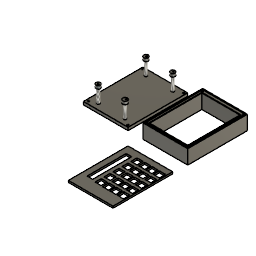
macropad-test-design (Autodesk Fusion 360 archive; units mm, degrees)
design "macropad-test-design"
part number: 2026-08-19-18-04-08-629
Autodesk Fusion 360 part; units mm, degrees
sketch "Sketch1" plane through (0, 0, 0) normal (0, 0, 1) x (1, 0, 0)
  line L0 (0, 100) -> (75, 100)
  line L1 (75, 100) -> (75, 0)
  line L2 (75, 0) -> (0, 0)
  line L3 (0, 0) -> (0, 100)
  line L4 (6.0568, 92.5343) -> (70, 92.5343)
  line L5 (70, 92.5343) -> (70, 5)
  line L6 (70, 5) -> (6.0568, 5)
  line L7 (6.0568, 5) -> (6.0568, 92.5343)
  constraint horizontal L0
  constraint vertical L1
  constraint horizontal L2
  constraint vertical L3
  constraint horizontal L4
  constraint vertical L5
  constraint horizontal L6
  constraint vertical L7
extrude "Extrude1" add sketch "Sketch1" along normal blind 20 makes body 1
sketch "Sketch2" plane through (0, 0, 0) normal (0, 0, 1) x (1, 0, 0)
  line L0 (-100, 100) -> (-25, 100)
  line L1 (-25, 100) -> (-25, 0)
  line L2 (-25, 0) -> (-100, 0)
  line L3 (-100, 0) -> (-100, 100)
  constraint horizontal L0
  constraint vertical L1
  constraint horizontal L2
  constraint vertical L3
extrude "Extrude2" add sketch "Sketch2" along normal blind 5 separate body makes body 2
cylinder "CylinderPrimitive1" add diameter 5 height 23 placed x (1, 0, 0) y (0, 1, 0) z (0, 0, 1) at (-40, 90, 5) bodies 2
cylinder "CylinderPrimitive2" add diameter 5 height 23 placed x (1, 0, 0) y (0, 1, 0) z (0, 0, 1) at (-85, 90, 5) bodies 2
cylinder "CylinderPrimitive3" add diameter 5 height 23 placed x (1, 0, 0) y (0, 1, 0) z (0, 0, 1) at (-85, 10, 5) bodies 2
cylinder "CylinderPrimitive4" add diameter 5 height 23 placed x (1, 0, 0) y (0, 1, 0) z (0, 0, 1) at (-40, 10, 5) bodies 2
extrude "Extrude3" add 1 faces at (27.0189, 97.5114, 20) along direction (0, 0, 1) blind 4 thin wall 1 inside on bodies 1 bodies 1
sketch "Sketch7" plane through (0, 0, 0) normal (0, 0, 1) x (1, 0, 0)
  line L0 (0, -25) -> (75, -25)
  line L1 (75, -25) -> (75, -125.149)
  line L2 (75, -125.149) -> (0, -125.149)
  line L3 (0, -125.149) -> (0, -25)
  constraint horizontal L0
  constraint vertical L1
  constraint horizontal L2
  constraint vertical L3
extrude "Extrude4" add sketch "Sketch7" along normal blind 3 separate body makes body 3
sketch "Sketch8" plane through (0, 0, 3) normal (0, 0, 1) x (-1, 0, 0)
  line L0 (0, 125.149) -> (-75, 125.149)
  line L1 (-75, 125.149) -> (-75, 25)
  line L2 (-75, 25) -> (0, 25)
  line L3 (0, 25) -> (0, 125.149)
  line L4 (-25, 35) -> (-35, 35)
  line L5 (-35, 35) -> (-35, 45)
  line L6 (-35, 45) -> (-25, 45)
  line L7 (-25, 45) -> (-25, 35)
  line L8 (-37.6867, 35) -> (-48.0057, 35)
  line L9 (-48.0057, 35) -> (-48.0057, 45)
  line L10 (-48.0057, 45) -> (-37.6867, 45)
  line L11 (-37.6867, 45) -> (-37.6867, 35)
  line L12 (-50, 35) -> (-60, 35)
  line L13 (-60, 35) -> (-60, 45)
  line L14 (-60, 45) -> (-50, 45)
  line L15 (-50, 45) -> (-50, 35)
  line L16 (-62.3625, 35) -> (-72.6815, 35)
  line L17 (-72.6815, 35) -> (-72.6815, 45)
  line L18 (-72.6815, 45) -> (-62.3625, 45)
  line L19 (-62.3625, 45) -> (-62.3625, 35)
  line L20 (-25, 50) -> (-35, 50)
  line L21 (-35, 50) -> (-35, 60)
  line L22 (-35, 60) -> (-25, 60)
  line L23 (-25, 60) -> (-25, 50)
  line L24 (-37.6867, 50) -> (-48.23, 50)
  line L25 (-48.23, 50) -> (-48.23, 60)
  line L26 (-48.23, 60) -> (-37.6867, 60)
  line L27 (-37.6867, 60) -> (-37.6867, 50)
  line L28 (-50, 50) -> (-60, 50)
  line L29 (-60, 50) -> (-60, 60)
  line L30 (-60, 60) -> (-50, 60)
  line L31 (-50, 60) -> (-50, 50)
  line L32 (-62.8111, 50) -> (-72.6815, 50)
  line L33 (-72.6815, 50) -> (-72.6815, 59.3341)
  line L34 (-72.6815, 59.3341) -> (-62.8111, 59.3341)
  line L35 (-62.8111, 59.3341) -> (-62.8111, 50)
  line L36 (-25, 65) -> (-35, 65)
  line L37 (-35, 65) -> (-35, 75)
  line L38 (-35, 75) -> (-25, 75)
  line L39 (-25, 75) -> (-25, 65)
  line L40 (-38.1353, 65) -> (-48.23, 65)
  line L41 (-48.23, 65) -> (-48.23, 75)
  line L42 (-48.23, 75) -> (-38.1353, 75)
  line L43 (-38.1353, 75) -> (-38.1353, 65)
  line L44 (-50, 65) -> (-60, 65)
  line L45 (-60, 65) -> (-60, 75)
  line L46 (-60, 75) -> (-50, 75)
  line L47 (-50, 75) -> (-50, 65)
  line L48 (-62.5868, 65) -> (-72.9058, 65)
  line L49 (-72.9058, 65) -> (-72.9058, 75)
  line L50 (-72.9058, 75) -> (-62.5868, 75)
  line L51 (-62.5868, 75) -> (-62.5868, 65)
  line L52 (-25, 80) -> (-35, 80)
  line L53 (-35, 80) -> (-35, 90)
  line L54 (-35, 90) -> (-25, 90)
  line L55 (-25, 90) -> (-25, 80)
  line L56 (-38.1353, 80) -> (-48.23, 80)
  line L57 (-48.23, 80) -> (-48.23, 90)
  line L58 (-48.23, 90) -> (-38.1353, 90)
  line L59 (-38.1353, 90) -> (-38.1353, 80)
  line L60 (-50, 80) -> (-60, 80)
  line L61 (-60, 80) -> (-60, 90)
  line L62 (-60, 90) -> (-50, 90)
  line L63 (-50, 90) -> (-50, 80)
  line L64 (-62.3625, 80) -> (-72.9058, 80)
  line L65 (-72.9058, 80) -> (-72.9058, 90)
  line L66 (-72.9058, 90) -> (-62.3625, 90)
  line L67 (-62.3625, 90) -> (-62.3625, 80)
  line L68 (-25, 95) -> (-35, 95)
  line L69 (-35, 95) -> (-35, 105)
  line L70 (-35, 105) -> (-25, 105)
  line L71 (-25, 105) -> (-25, 95)
  line L72 (-37.6867, 95) -> (-47.6867, 95)
  line L73 (-47.6867, 95) -> (-47.6867, 105.5451)
  line L74 (-47.6867, 105.5451) -> (-37.6867, 105.5451)
  line L75 (-37.6867, 105.5451) -> (-37.6867, 95)
  line L76 (-50, 95) -> (-60.1192, 95)
  line L77 (-60.1192, 95) -> (-60.1192, 105.5451)
  line L78 (-60.1192, 105.5451) -> (-50, 105.5451)
  line L79 (-50, 105.5451) -> (-50, 95)
  line L80 (-62.5868, 95) -> (-72.9058, 95)
  line L81 (-72.9058, 95) -> (-72.9058, 105.5451)
  line L82 (-72.9058, 105.5451) -> (-62.5868, 105.5451)
  line L83 (-62.5868, 105.5451) -> (-62.5868, 95)
  line L84 (-30, 40) -> (-28.7137, 40)
  line L85 (-28.7137, 40) -> (-28.7137, 37.7988)
  line L86 (-28.7137, 37.7988) -> (-30, 37.7988)
  line L87 (-30, 37.7988) -> (-30, 40)
  dimension "d18" = 10
  constraint horizontal L4
  constraint vertical L5
  constraint horizontal L6
  constraint vertical L7
  constraint horizontal L8
  constraint vertical L9
  constraint horizontal L10
  constraint vertical L11
  constraint horizontal L12
  constraint vertical L13
  constraint horizontal L14
  constraint vertical L15
  constraint horizontal L16
  constraint vertical L17
  constraint horizontal L18
  constraint vertical L19
  constraint horizontal L20
  constraint vertical L21
  constraint horizontal L22
  constraint vertical L23
  constraint horizontal L24
  constraint vertical L25
  constraint horizontal L26
  constraint vertical L27
  constraint horizontal L28
  constraint vertical L29
  constraint horizontal L30
  constraint vertical L31
  constraint horizontal L32
  constraint vertical L33
  constraint horizontal L34
  constraint vertical L35
  constraint horizontal L36
  constraint vertical L37
  constraint horizontal L38
  constraint vertical L39
  constraint horizontal L40
  constraint vertical L41
  constraint horizontal L42
  constraint vertical L43
  constraint horizontal L44
  constraint vertical L45
  constraint horizontal L46
  constraint vertical L47
  constraint horizontal L48
  constraint vertical L49
  constraint horizontal L50
  constraint vertical L51
  constraint horizontal L52
  constraint vertical L53
  constraint horizontal L54
  constraint vertical L55
  constraint horizontal L56
  constraint vertical L57
  constraint horizontal L58
  constraint vertical L59
  constraint horizontal L60
  constraint vertical L61
  constraint horizontal L62
  constraint vertical L63
  constraint horizontal L64
  constraint vertical L65
  constraint horizontal L66
  constraint vertical L67
  constraint horizontal L68
  constraint vertical L69
  constraint horizontal L70
  constraint vertical L71
  constraint horizontal L72
  constraint vertical L73
  constraint horizontal L74
  constraint vertical L75
  constraint horizontal L76
  constraint vertical L77
  constraint horizontal L78
  constraint vertical L79
  constraint horizontal L80
  constraint vertical L81
  constraint horizontal L82
  constraint vertical L83
  constraint horizontal L84
  constraint vertical L85
  constraint horizontal L86
  constraint vertical L87
  measures "d18" distance of L72.start L72.end
extrude "Extrude5" cut sketch "Sketch8" against normal blind 5 contours L4 L5 L6 L7 | L8 L9 L10 L11 | L12 L13 L14 L15 | L16 L17 L18 L19 | L20 L21 L22 L23 | L24 L25 L26 L27 | L28 L29 L30 L31 | L32 L33 L34 L35 | L36 L37 L38 L39 | L40 L41 L42 L43 | L44 L45 L46 L47 | L48 L49 L50 L51 | L52 L53 L54 L55 | L56 L57 L58 L59 | L60 L61 L62 L63 | L64 L65 L66 L67 | L68 L69 L70 L71 | L72 L73 L74 L75 | L76 L77 L78 L79 | L80 L81 L82 L83 | L84 L85 L86 L87 bodies 3
sketch "Sketch9" plane through (0, 0, 0) normal (0, 0, 1) x (1, 0, 0)
thread "Thread1" "ISO Metric profile 4.5 M4.5x0.75 M4.5x0.75 6g" major diameter 4.408 minor diameter 3.5525 pitch 0.75 angle 60 resizes the face on face at (-42.3037, 89.0289, 12.6667) on bodies 2
thread "Thread2" "ISO Metric profile 4.5 M4.5x0.75 M4.5x0.75 6g" major diameter 4.408 minor diameter 3.5525 pitch 0.75 angle 60 resizes the face on face at (-87.3037, 89.0289, 12.6667) on bodies 2
thread "Thread3" "ISO Metric profile 5.0 M5x0.8 M5x0.8 6g" major diameter 4.901 minor diameter 3.9895 pitch 0.8 angle 60 resizes the face on face at (-82.5124, 9.7511, 20.3333) on bodies 2
cylinder "CylinderPrimitive5" add diameter 8 height 5 placed x (1, 0, 0) y (0, 1, 0) z (0, 0, 1) at (-40, 90, 28) bodies 2
cylinder "CylinderPrimitive6" add diameter 8 height 5 placed x (1, 0, 0) y (0, 1, 0) z (0, 0, 1) at (-85, 90, 28) bodies 2
cylinder "CylinderPrimitive7" add diameter 8 height 5 placed x (1, 0, 0) y (0, 1, 0) z (0, 0, 1) at (-40, 10, 28) bodies 2
sketch "Sketch13" plane through (0, 0, 28) normal (0, 0, 1) x (-1, 0, 0)
  circle A0 centre (85, -10) radius 2.4505
hole "Hole1" at (-40.0298, 90.0437, 33) direction (0, 0, -1) diameter 0.19 depth 2.4 tip angle 118 bodies 2
thread "Thread4" "ISO Metric profile 0.25 M0.25x0.075 M0.25x0.075 6H" thread offset 0 thread depth 7.4
hole "Hole2" at (-84.8949, 90.0437, 33) direction (0, 0, -1) diameter 0.19 depth 2.4 tip angle 118 bodies 2
thread "Thread5" "ISO Metric profile 0.25 M0.25x0.075 M0.25x0.075 6H" thread offset 0 thread depth 7.4
cylinder "CylinderPrimitive8" add diameter 8 height 5 placed x (1, 0, 0) y (0, 1, 0) z (0, 0, 1) at (-85, 10, 28) bodies 2
hole "Hole3" at (-84.8949, 9.7352, 33) direction (0, 0, -1) diameter 0.19 depth 2.4 tip angle 118 counterbore diameter 2.4 counterbore depth 1 bodies 2
thread "Thread6" "ISO Metric profile 0.25 M0.25x0.075 M0.25x0.075 6H" thread offset 0 thread depth 2.4
hole "Hole4" at (-84.5438, 90.5438, 33) direction (0, 0, -1) diameter 0.19 depth 10 tip angle 118 counterbore diameter 2.4 counterbore depth 1 bodies 2
thread "Thread7" "ISO Metric profile 0.25 M0.25x0.075 M0.25x0.075 6H" thread offset 0 thread depth 2.16
hole "Hole5" at (-39.2616, 90.4676, 33) direction (0, 0, -1) diameter 0.19 depth 5 tip angle 118 counterbore diameter 2.4 counterbore depth 4.5 bodies 2
thread "Thread8" "ISO Metric profile 0.25 M0.25x0.075 M0.25x0.075 6H" thread offset 0 thread depth 4.5
thread "Thread9" "ISO Metric profile 4.5 M4.5x0.75 M4.5x0.75 6g" major diameter 4.408 minor diameter 3.5525 pitch 0.75 angle 60 resizes the face on face at (-37.5124, 9.7511, 20.3333) on bodies 2
hole "Hole6" at (-39.5298, 11.5445, 33) direction (0, 0, -1) diameter 0.19 depth 5 tip angle 118 counterbore diameter 2.4 counterbore depth 1 bodies 2
thread "Thread10" "ISO Metric profile 0.25 M0.25x0.075 M0.25x0.075 6H" thread offset 0 thread depth 4.5
sketch "Sketch15" plane through (0, 0, 3) normal (0, 0, 1) x (-1, 0, 0)
  line L0 (0, 125.149) -> (-75, 125.149)
  line L1 (-75, 125.149) -> (-75, 25)
  line L2 (-75, 25) -> (0, 25)
  line L3 (0, 25) -> (0, 125.149)
  line L4 (-60, 50) -> (-60, 60)
  line L5 (-60, 60) -> (-50, 60)
  line L6 (-50, 60) -> (-50, 50)
  line L7 (-50, 50) -> (-60, 50)
  line L8 (-48.0057, 35) -> (-48.0057, 45)
  line L9 (-48.0057, 45) -> (-37.6867, 45)
  line L10 (-37.6867, 45) -> (-37.6867, 35)
  line L11 (-37.6867, 35) -> (-48.0057, 35)
  line L12 (-35, 65) -> (-35, 75)
  line L13 (-35, 75) -> (-25, 75)
  line L14 (-25, 75) -> (-25, 65)
  line L15 (-25, 65) -> (-35, 65)
  line L16 (-35, 80) -> (-35, 90)
  line L17 (-35, 90) -> (-25, 90)
  line L18 (-25, 90) -> (-25, 80)
  line L19 (-25, 80) -> (-35, 80)
  line L20 (-60, 65) -> (-60, 75)
  line L21 (-60, 75) -> (-50, 75)
  line L22 (-50, 75) -> (-50, 65)
  line L23 (-50, 65) -> (-60, 65)
  line L24 (-60.1192, 95) -> (-60.1192, 105.5451)
  line L25 (-60.1192, 105.5451) -> (-50, 105.5451)
  line L26 (-50, 105.5451) -> (-50, 95)
  line L27 (-50, 95) -> (-60.1192, 95)
  line L28 (-72.6815, 50) -> (-72.6815, 59.3341)
  line L29 (-72.6815, 59.3341) -> (-62.8111, 59.3341)
  line L30 (-62.8111, 59.3341) -> (-62.8111, 50)
  line L31 (-62.8111, 50) -> (-72.6815, 50)
  line L32 (-48.23, 80) -> (-48.23, 90)
  line L33 (-48.23, 90) -> (-38.1353, 90)
  line L34 (-38.1353, 90) -> (-38.1353, 80)
  line L35 (-38.1353, 80) -> (-48.23, 80)
  line L36 (-35, 95) -> (-35, 105)
  line L37 (-35, 105) -> (-25, 105)
  line L38 (-25, 105) -> (-25, 95)
  line L39 (-25, 95) -> (-35, 95)
  line L40 (-35, 50) -> (-35, 60)
  line L41 (-35, 60) -> (-25, 60)
  line L42 (-25, 60) -> (-25, 50)
  line L43 (-25, 50) -> (-35, 50)
  line L44 (-72.6815, 35) -> (-72.6815, 45)
  line L45 (-72.6815, 45) -> (-62.3625, 45)
  line L46 (-62.3625, 45) -> (-62.3625, 35)
  line L47 (-62.3625, 35) -> (-72.6815, 35)
  line L48 (-72.9058, 95) -> (-72.9058, 105.5451)
  line L49 (-72.9058, 105.5451) -> (-62.5868, 105.5451)
  line L50 (-62.5868, 105.5451) -> (-62.5868, 95)
  line L51 (-62.5868, 95) -> (-72.9058, 95)
  line L52 (-48.23, 50) -> (-48.23, 60)
  line L53 (-48.23, 60) -> (-37.6867, 60)
  line L54 (-37.6867, 60) -> (-37.6867, 50)
  line L55 (-37.6867, 50) -> (-48.23, 50)
  line L56 (-60, 80) -> (-60, 90)
  line L57 (-60, 90) -> (-50, 90)
  line L58 (-50, 90) -> (-50, 80)
  line L59 (-50, 80) -> (-60, 80)
  line L60 (-72.9058, 65) -> (-72.9058, 75)
  line L61 (-72.9058, 75) -> (-62.5868, 75)
  line L62 (-62.5868, 75) -> (-62.5868, 65)
  line L63 (-62.5868, 65) -> (-72.9058, 65)
  line L64 (-48.23, 65) -> (-48.23, 75)
  line L65 (-48.23, 75) -> (-38.1353, 75)
  line L66 (-38.1353, 75) -> (-38.1353, 65)
  line L67 (-38.1353, 65) -> (-48.23, 65)
  line L68 (-35, 35) -> (-35, 45)
  line L69 (-35, 45) -> (-25, 45)
  line L70 (-25, 45) -> (-25, 35)
  line L71 (-25, 35) -> (-35, 35)
  line L72 (-72.9058, 80) -> (-72.9058, 90)
  line L73 (-72.9058, 90) -> (-62.3625, 90)
  line L74 (-62.3625, 90) -> (-62.3625, 80)
  line L75 (-62.3625, 80) -> (-72.9058, 80)
  line L76 (-47.6867, 95) -> (-47.6867, 105.5451)
  line L77 (-47.6867, 105.5451) -> (-37.6867, 105.5451)
  line L78 (-37.6867, 105.5451) -> (-37.6867, 95)
  line L79 (-37.6867, 95) -> (-47.6867, 95)
  line L80 (-60, 35) -> (-60, 45)
  line L81 (-60, 45) -> (-50, 45)
  line L82 (-50, 45) -> (-50, 35)
  line L83 (-50, 35) -> (-60, 35)
  line L84 (-9.5689, 37.7439) -> (-18.7125, 37.7439)
  line L85 (-18.7125, 37.7439) -> (-18.7125, 103.025)
  line L86 (-18.7125, 103.025) -> (-9.5689, 103.025)
  line L87 (-9.5689, 103.025) -> (-9.5689, 37.7439)
  constraint horizontal L84
  constraint vertical L85
  constraint horizontal L86
  constraint vertical L87
extrude "Extrude6" cut sketch "Sketch15" against normal blind 3 contours L84 L85 L86 L87 bodies 3
sketch "Sketch16" plane through (0, 0, 0) normal (0, 0, 1) x (1, 0, 0)
  line L0 (116.3152, -42.2094) -> (123.545, -42.2094)
  line L1 (123.545, -42.2094) -> (123.545, -48.376)
  line L2 (123.545, -48.376) -> (116.3152, -48.376)
  line L3 (116.3152, -48.376) -> (116.3152, -42.2094)
  constraint horizontal L0
  constraint vertical L1
  constraint horizontal L2
  constraint vertical L3
sketch "Sketch17" plane through (123.545, 0, 0) normal (-1, 0, 0) x (0, -1, 0)
extrude "Extrude8" add 1 faces at (26.6856, 97.1781, 20) along direction (0, 0, 1) blind 3 on bodies 1 bodies 1
hole "Hole7" at (3.2584, 3.1008, 23) direction (0, 0, -1) diameter 3 depth 30 tip angle 180 bodies 1
hole "Hole8" at (72.0341, 2.9659, 23) direction (0, 0, -1) diameter 3 depth 30 tip angle 180 bodies 1
hole "Hole9" at (71.4699, 96.238, 23) direction (0, 0, -1) diameter 3 depth 30 tip angle 180 bodies 1
hole "Hole10" at (3.4383, 95.6923, 23) direction (0, 0, -1) diameter 3 depth 30 tip angle 180 bodies 1
hole "Hole11" at (-96.1311, 4.7426, 5) direction (0, 0, -1) diameter 3 depth 2 tip angle 180 bodies 2
hole "Hole12" at (-28.2449, 2.9953, 5) direction (0, 0, -1) diameter 3 depth 2 tip angle 180 bodies 2
hole "Hole13" at (-27.9953, 96.5055, 5) direction (0, 0, -1) diameter 3 depth 2 tip angle 180 bodies 2
hole "Hole14" at (-97.3791, 96.7551, 5) direction (0, 0, -1) diameter 2.4 depth 2 tip angle 180 bodies 2
